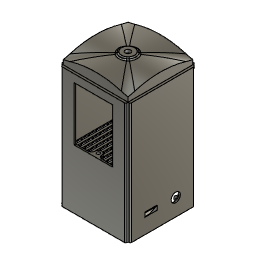
SolderingStation_Front (Autodesk Fusion 360 design; units mm, degrees)
Autodesk Fusion 360 part; units mm, degrees
sketch "Sketch1" plane through (0, 0, 0) normal (0, 0, 1) x (1, 0, 0)
  line L0 (45, 45) -> (-45, 45)
  line L1 (-45, 45) -> (-45, -45)
  line L2 (-45, -45) -> (45, -45)
  line L3 (45, -45) -> (45, 45)
  line L4 (45, 45) -> (-45, -45) construction
  line L5 (-45, 45) -> (45, -45) construction
  line L6 (0, 0) -> (0, -45) construction
  line L7 (0, 0) -> (-45, 0) construction
  line L8 (-45, -45) -> (-42, -45) construction
  line L9 (-42, -45) -> (-42, -42)
  line L10 (-45, -42) -> (-42, -42)
  line L11 (45, -42) -> (42, -42)
  line L12 (42, -45) -> (42, -42)
  line L13 (42, 45) -> (42, 42)
  line L14 (45, 42) -> (42, 42)
  line L15 (-45, 42) -> (-42, 42)
  line L16 (-42, 45) -> (-42, 42)
  dimension "d1" = 90
  dimension "d2" = 90
  dimension "d10" = 360
  constraint horizontal L0
  constraint perpendicular L0 L1
  constraint parallel L0 L2
  constraint parallel L1 L3
  constraint coincident L4 L6.start
  constraint coincident L5 L6.start
  constraint coincident L6.start L7.start
  constraint midpoint L2 L6.end
  constraint midpoint L1 L7.end
  constraint coincident L2 L8.end
  constraint coincident L4 L9.end
  constraint perpendicular L2 L9
  constraint perpendicular L9 L10
  measures "d1" distance of L1.end L2.end
  measures "d2" distance of L0.end L1.end
extrude "Extrude3" add sketch "Sketch1" along normal blind 2 contours L0 L1 L2 L3 L9 L10 L11 L12 L13 L14 L15 L16 makes body 1
sketch "Sketch3" plane through (0, 0, 0) normal (0, 0, -1) x (1, 0, 0)
  line L0 (-42, -45) -> (42, -45)
  line L1 (42, -45) -> (42, -42)
  line L2 (42, -42) -> (45, -42)
  line L3 (45, -42) -> (45, 42)
  line L4 (45, 42) -> (42, 42)
  line L5 (42, 42) -> (42, 45)
  line L6 (42, 45) -> (-42, 45)
  line L7 (-42, 45) -> (-42, 42)
  line L8 (-42, 42) -> (-45, 42)
  line L9 (-45, 42) -> (-45, -42)
  line L10 (-45, -42) -> (-42, -42)
  line L11 (-42, -42) -> (-42, -45)
  line L12 (43, -42) -> (43, 40)
  line L13 (43, 40) -> (40, 40)
  line L14 (40, 40) -> (40, 43)
  line L15 (40, 43) -> (-40, 43)
  line L16 (-40, 43) -> (-40, 40)
  line L17 (-40, 40) -> (-43, 40)
  line L18 (-43, 40) -> (-43, -42)
  line L19 (-45, -42) -> (-45, -40) construction
  line L20 (-45, -40) -> (-43, -40)
  line L21 (43, -40) -> (45, -40)
  dimension "d13" = -2
  constraint coincident L9.end L10.start
  constraint coincident L9 L19.end
  constraint perpendicular L10 L19
  constraint coincident L18 L20.end
  constraint perpendicular L18 L20
  constraint coincident L12 L21.start
  constraint coincident L3 L21.end
  constraint perpendicular L3 L21
extrude "Extrude4" add sketch "Sketch3" along normal blind 155 contours L3 L4 L5 L6 L7 L8 L9 L12 L13 L14 L15 L16 L17 L18 L20 L21 bodies 1
sketch "Sketch4" plane through (0, 40, 0) normal (0, 1, 0) x (-1, 0, 0)
  line L0 (45, 0) -> (43, 0)
  line L1 (43, 0) -> (43, -155)
  line L2 (43, -155) -> (45, -155)
  line L3 (45, -155) -> (45, 0)
  line L4 (43, -155) -> (43, -145) construction
  line L5 (43, -145) -> (37, -145) construction
  circle A0 centre (37, -145) radius 2.15
  circle A1 centre (37, -145) radius 4.5
  line L6 (37, -145) -> (37, -140.5) construction
  line L7 (37, -145) -> (37, -149.5) construction
  line L8 (37, -149.5) -> (43, -149.5)
  line L9 (37, -140.5) -> (43, -140.5)
  line L10 (0, -155) -> (0, 2) construction
  line L11 (-37, -140.5) -> (-43, -140.5)
  circle A2 centre (-37, -145) radius 4.5
  circle A3 centre (-37, -145) radius 2.15
  line L12 (-37, -149.5) -> (-43, -149.5)
  circle A4 centre (37, -5) radius 4.5
  circle A5 centre (37, -5) radius 2.15
  line L13 (37, -9.5) -> (43, -9.5)
  line L14 (37, -0.5) -> (43, -0.5)
  line L15 (-37, -0.5) -> (-43, -0.5)
  circle A6 centre (-37, -5) radius 4.5
  circle A7 centre (-37, -5) radius 2.15
  line L16 (-37, -9.5) -> (-43, -9.5)
  line L17 (-43, -140.5) -> (-43, -149.5)
  line L18 (-43, -0.5) -> (-43, -9.5)
  dimension "d16" = 4.3
  dimension "d17" = 9
  dimension "d18" = 4.3
  dimension "d19" = 9
  constraint coincident L1.end L2.start
  constraint coincident L1 L4.end
  constraint perpendicular L2 L4
  constraint perpendicular L4 L5
  constraint coincident L5.end A0.centre
  constraint concentric A0 A1
  constraint coincident A1 L6.end
  constraint perpendicular L5 L6
  constraint coincident A1 L7.end
  constraint perpendicular L5 L7
  constraint coincident L4 L8.end
  constraint coincident L1 L9.end
  constraint tangent A1 L9
  constraint perpendicular L9 L10
  constraint symmetric A0 L10 A3
  constraint symmetric A1 L10 A2
  constraint symmetric L6.end L10 L11.start
  constraint symmetric L7.end L10 L12.start
  constraint symmetric L8.end L10 L12.end
  constraint symmetric L9.end L10 L11.end
  constraint concentric A4 A5
  constraint coincident L14.start A4
  constraint coincident L13.start A4
  constraint tangent A4 L14
  constraint vertical L18
  measures "d16" diameter of A0
  measures "d17" diameter of A1
  measures "d18" diameter of A5
  measures "d19" diameter of A4
extrude "Extrude5" add sketch "Sketch4" against normal blind 13 contours L1 A4 L13 L14 | A4 | L1 A1 L8 L9 | A1 | L11 A2 L12 L17 | A2 | L15 A6 L16 L18 | A6 bodies 1
ref_plane "WorkPlane1" through (0, 35, 0) normal (0, 1, 0) x (0, 0, 1)
sketch "Sketch5" plane through (0, 35, 0) normal (0, 1, 0) x (1, 0, 0)
  circle A0 centre (37, 5) radius 2.15 construction
  line L0 (0, -2) -> (0, 155) construction
  line L1 (35.0226, 8.425) -> (33.0452, 5)
  line L2 (33.0452, 5) -> (35.0226, 1.575)
  line L3 (35.0226, 1.575) -> (38.9774, 1.575)
  line L4 (38.9774, 1.575) -> (40.9548, 5)
  line L5 (40.9548, 5) -> (38.9774, 8.425)
  line L6 (38.9774, 8.425) -> (35.0226, 8.425)
  line L7 (35.0226, 1.575) -> (31.6368, 1.575)
  line L8 (35.0226, 8.425) -> (31.5846, 8.425)
  line L9 (31.5846, 8.425) -> (31.6368, 1.575)
  line L10 (-35.0226, 1.575) -> (-38.9774, 1.575)
  line L11 (-38.9774, 1.575) -> (-40.9548, 5)
  line L12 (-40.9548, 5) -> (-38.9774, 8.425)
  line L13 (-38.9774, 8.425) -> (-35.0226, 8.425)
  line L14 (-35.0226, 8.425) -> (-31.5846, 8.425)
  line L15 (-31.5846, 8.425) -> (-31.6368, 1.575)
  line L16 (-35.0226, 1.575) -> (-31.6368, 1.575)
  line L17 (-33.0452, 5) -> (-35.0226, 1.575)
  line L18 (-35.0226, 8.425) -> (-33.0452, 5)
  line L19 (35.0226, 141.575) -> (38.9774, 141.575)
  line L20 (33.0452, 145) -> (35.0226, 141.575)
  line L21 (38.9774, 141.575) -> (40.9548, 145)
  line L22 (40.9548, 145) -> (38.9774, 148.425)
  line L23 (38.9774, 148.425) -> (35.0226, 148.425)
  line L24 (35.0226, 148.425) -> (31.5846, 148.425)
  line L25 (35.0226, 148.425) -> (33.0452, 145)
  line L26 (31.5846, 148.425) -> (31.6368, 141.575)
  line L27 (35.0226, 141.575) -> (31.6368, 141.575)
  line L28 (-38.9774, 141.575) -> (-40.9548, 145)
  line L29 (-35.0226, 141.575) -> (-38.9774, 141.575)
  line L30 (-35.0226, 141.575) -> (-31.6368, 141.575)
  line L31 (-31.5846, 148.425) -> (-31.6368, 141.575)
  line L32 (-35.0226, 148.425) -> (-31.5846, 148.425)
  line L33 (-35.0226, 148.425) -> (-33.0452, 145)
  line L34 (-33.0452, 145) -> (-35.0226, 141.575)
  line L35 (-38.9774, 148.425) -> (-35.0226, 148.425)
  line L36 (-40.9548, 145) -> (-38.9774, 148.425)
  point P0 (37, 5)
  dimension "d24" = 4.3
  dimension "d25" = 3.425
  constraint vertical L0
  constraint coincident P0 A0.centre
  constraint parallel L3 L7
  constraint parallel L6 L8
  constraint symmetric L0 L1.start L13.end
  constraint symmetric L0 L1.end L17.start
  constraint symmetric L0 L2.end L10.start
  constraint symmetric L0 L3.end L10.end
  constraint symmetric L0 L4.end L11.end
  constraint symmetric L0 L5.end L12.end
  constraint symmetric L0 L7.end L15.end
  constraint symmetric L0 L8.end L14.end
  constraint parallel L19 L27
  constraint parallel L23 L24
  measures "d24" diameter of A0
  measures "d25" distance of P0 L6
extrude "Extrude6" cut sketch "Sketch5" against normal blind 3 bodies 1
sketch "Sketch6" plane through (0, -45, 0) normal (0, -1, 0) x (1, 0, 0)
  line L0 (42, -155) -> (42, 2)
  line L1 (42, 2) -> (-42, 2)
  line L2 (-42, 2) -> (-42, -155)
  line L3 (-42, -155) -> (42, -155)
  line L4 (0, 2) -> (0, -155) construction
  line L5 (25, -8) -> (-25, -8)
  line L6 (-25, -8) -> (-25, -78)
  line L7 (-25, -78) -> (25, -78)
  line L8 (25, -78) -> (25, -8)
  line L9 (25, -8) -> (-25, -78) construction
  line L10 (-25, -8) -> (25, -78) construction
  point P0 (0, -43)
  dimension "d28" = 70
  dimension "d29" = 50
  dimension "d30" = 45
  constraint midpoint L1 L4.start
  constraint midpoint L3 L4.end
  constraint horizontal L5
  constraint perpendicular L5 L6
  constraint parallel L5 L7
  constraint parallel L6 L8
  constraint coincident L9 P0
  constraint coincident L10 P0
  constraint coincident L4 P0
  measures "d28" distance of L5.start L7.end
  measures "d29" distance of L5.start L5.end
  measures "d30" distance of L1 P0
extrude "Extrude7" cut sketch "Sketch6" against normal blind 2 contours L5 L6 L7 L8 bodies 1
sketch "Sketch7" plane through (0, -45, 0) normal (0, -1, 0) x (1, 0, 0)
  line L0 (-25, -8) -> (25, -8)
  line L1 (25, -8) -> (25, -78)
  line L2 (25, -78) -> (-25, -78)
  line L3 (-25, -78) -> (-25, -8)
  line L4 (42, -155) -> (42, 2)
  line L5 (42, 2) -> (-42, 2)
  line L6 (-42, 2) -> (-42, -155)
  line L7 (-42, -155) -> (42, -155)
  line L8 (0, 2) -> (0, -155) construction
  line L9 (4.5, -8) -> (-4.5, -8)
  line L10 (-4.5, -8) -> (-4.5, -5)
  line L11 (-4.5, -5) -> (4.5, -5)
  line L12 (4.5, -5) -> (4.5, -8)
  line L13 (25, -43) -> (-25, -43) construction
  line L14 (-4.5, -81) -> (4.5, -81)
  line L15 (4.5, -78) -> (-4.5, -78)
  line L16 (-4.5, -78) -> (-4.5, -81)
  line L17 (4.5, -81) -> (4.5, -78)
  dimension "d35" = 9
  dimension "d36" = 3
  dimension "d37" = 4.5
  constraint midpoint L5 L8.start
  constraint midpoint L7 L8.end
  constraint horizontal L9
  constraint vertical L10
  constraint horizontal L11
  constraint vertical L12
  constraint midpoint L1 L13.start
  constraint midpoint L3 L13.end
  constraint symmetric L9.start L13 L15.start
  constraint symmetric L9.end L13 L15.end
  constraint symmetric L10.end L13 L14.start
  constraint symmetric L11.end L13 L14.end
  measures "d35" distance of L9.start L9.end
  measures "d36" distance of L9.start L11.end
  measures "d37" distance of L8 L12
extrude "Extrude8" add sketch "Sketch7" against normal blind 11 contours L0 L9 L10 L11 L12 | L2 L14 L15 L16 L17 bodies 1
sketch "Sketch9" plane through (0, 0, -81) normal (0, 0, -1) x (1, 0, 0)
  line L0 (4.5, 43) -> (-4.5, 43)
  line L1 (-4.5, 43) -> (-4.5, 34)
  line L2 (-4.5, 34) -> (4.5, 34)
  line L3 (4.5, 34) -> (4.5, 43)
  line L4 (-4.5, 43) -> (4.5, 34) construction
  line L5 (-4.5, 34) -> (4.5, 43) construction
  circle A0 centre (0, 38.5) radius 2.15
  dimension "d40" = 4.3
  constraint coincident L0.end L1.start
  constraint coincident L2.end L3.start
  constraint coincident L1.end L2.start
  constraint coincident L0.start L3.end
  constraint midpoint L5 A0.centre
  measures "d40" diameter of A0
extrude "Extrude9" cut sketch "Sketch9" against normal blind 80 contours A0 bodies 1
fillet "Fillet1" radius 4.5 8 edges at (4.5, -34, -79.5) (-4.5, -34, -79.5) (4.5, -43, -79.5) (-4.5, -43, -79.5) (4.5, -34, -6.5) (-4.5, -34, -6.5) (4.5, -43, -6.5) (-4.5, -43, -6.5) on bodies 1
sketch "Sketch10" plane through (0, 0, -155) normal (0, 0, -1) x (1, 0, 0)
  line L0 (43, 40) -> (43, -40)
  line L1 (43, -40) -> (45, -40)
  line L2 (45, -40) -> (45, 42)
  line L3 (45, 42) -> (42, 42)
  line L4 (42, 42) -> (42, 45)
  line L5 (42, 45) -> (-42, 45)
  line L6 (-42, 45) -> (-42, 42)
  line L7 (-42, 42) -> (-45, 42)
  line L8 (-45, 42) -> (-45, -40)
  line L9 (-45, -40) -> (-43, -40)
  line L10 (-43, -40) -> (-43, 40)
  line L11 (-43, 40) -> (-40, 40)
  line L12 (-40, 40) -> (-40, 43)
  line L13 (-40, 43) -> (40, 43)
  line L14 (40, 43) -> (40, 40)
  line L15 (40, 40) -> (43, 40)
  line L16 (0, 0) -> (0, 45) construction
  circle A0 centre (-36.452, 36.452) radius 2.15
  circle A1 centre (-36.452, 36.452) radius 4.5
  line L17 (-36.452, 36.452) -> (-31.952, 36.452) construction
  line L18 (-36.452, 36.452) -> (-36.452, 31.952) construction
  line L19 (-31.952, 36.452) -> (-31.952, 45)
  line L20 (-36.452, 31.952) -> (-45, 31.952)
  line L21 (31.952, 36.452) -> (31.952, 45)
  circle A2 centre (36.452, 36.452) radius 4.5
  circle A3 centre (36.452, 36.452) radius 2.15
  line L22 (36.452, 31.952) -> (45, 31.952)
  dimension "d45" = 4.3
  dimension "d46" = 8.548
  dimension "d47" = 8.548
  dimension "d48" = 9
  constraint coincident L16.start origin
  constraint midpoint L5 L16.end
  constraint concentric A0 A1
  constraint coincident A0.centre A1.centre
  constraint coincident A1 L17.end
  constraint parallel L13 L17
  constraint coincident A1 L18.end
  constraint perpendicular L17 L18
  constraint coincident L5 L19.end
  constraint tangent A1 L19
  constraint tangent A1 L20
  constraint symmetric L16 A0 A3
  constraint symmetric L16 A1 A2
  constraint symmetric L16 L17.end L21.start
  constraint symmetric L16 L18.end L22.start
  constraint symmetric L16 L19.end L21.end
  constraint symmetric L16 L20.end L22.end
  measures "d45" diameter of A0
  measures "d46" distance of L5 A0.centre
  measures "d47" distance of L8 A0.centre
  measures "d48" diameter of A1
extrude "Extrude10" add sketch "Sketch10" against normal blind 13 contours L0 L13 L14 L15 L21 A2 L22 | A2 | L10 L11 L12 L13 A1 L19 L20 | A1 bodies 1
ref_plane "WorkPlane2" through (0, 0, -150) normal (0, 0, 1) x (1, 0, 0)
sketch "Sketch11" plane through (0, 0, -150) normal (0, 0, 1) x (1, 0, 0)
  circle A0 centre (-36.454, -36.454) radius 2.15 construction
  line L0 (42, -45) -> (-42, -45) construction
  line L1 (-45, -42) -> (-45, 40) construction
  line L2 (0, -45) -> (0, 0) construction
  line L3 (-39.879, -38.4314) -> (-36.454, -40.4088)
  line L4 (-36.454, -40.4088) -> (-33.029, -38.4314)
  line L5 (-33.029, -38.4314) -> (-33.029, -34.4766)
  line L6 (-33.029, -34.4766) -> (-36.454, -32.4992)
  line L7 (-36.454, -32.4992) -> (-39.879, -34.4766)
  line L8 (-39.879, -34.4766) -> (-39.879, -38.4314)
  line L9 (-39.879, -34.4766) -> (-39.879, -31.1512)
  line L10 (-33.029, -34.4766) -> (-33.029, -31)
  line L11 (-33.029, -31) -> (-39.879, -31.1512)
  line L12 (33.029, -38.4314) -> (33.029, -34.4766)
  line L13 (36.454, -40.4088) -> (33.029, -38.4314)
  line L14 (39.879, -38.4314) -> (36.454, -40.4088)
  line L15 (39.879, -34.4766) -> (39.879, -38.4314)
  line L16 (36.454, -32.4992) -> (39.879, -34.4766)
  line L17 (33.029, -34.4766) -> (36.454, -32.4992)
  line L18 (33.029, -31) -> (39.879, -31.1512)
  line L19 (33.029, -34.4766) -> (33.029, -31)
  line L20 (39.879, -34.4766) -> (39.879, -31.1512)
  point P0 (-36.454, -36.454)
  dimension "d52" = 4.3
  dimension "d53" = 8.546
  dimension "d54" = 8.546
  dimension "d55" = 3.425
  constraint midpoint L0 L2.start
  constraint coincident L2.end origin
  constraint coincident P0 A0.centre
  constraint parallel L8 L9
  constraint parallel L5 L10
  constraint symmetric L2 L3.start L14.start
  constraint symmetric L2 L3.end L13.start
  constraint symmetric L2 L4.end L12.start
  constraint symmetric L2 L5.end L12.end
  constraint symmetric L2 L6.end L16.start
  constraint symmetric L2 L7.end L15.start
  constraint symmetric L2 L9.end L18.end
  constraint symmetric L2 L10.end L18.start
  measures "d52" diameter of A0
  measures "d53" distance of P0 L0
  measures "d54" distance of P0 L1
  measures "d55" distance of P0 L8
extrude "Extrude11" cut sketch "Sketch11" against normal blind 3 bodies 1
ref_plane "WorkPlane3" through (0, -25, 0) normal (0, 1, 0) x (0, 0, 1)
sketch "Sketch13" plane through (0, -25, 0) normal (0, 1, 0) x (1, 0, 0)
  line L0 (43, 138.3124) -> (37.453, 146.6329)
  line L1 (43, 138.3124) -> (53, 138.3124) construction
  line L2 (37.453, 146.6329) -> (34.7904, 144.8578)
  line L3 (43, 138.3124) -> (43, 124) construction
  line L4 (34.7904, 144.8578) -> (43, 132.5435)
  line L5 (44.6641, 139.4218) -> (38.0077, 149.4064)
  line L6 (38.0077, 149.4064) -> (32.0169, 145.4125)
  line L7 (32.0169, 145.4125) -> (41.3359, 131.4341)
  line L8 (41.3359, 131.4341) -> (43, 128.9379)
  line L9 (43, 138.3124) -> (43, 151) construction
  line L10 (38.0077, 149.4064) -> (43, 149.4064)
  line L11 (43, 128.9379) -> (43, 141.9179)
  line L12 (38.0077, 149.4064) -> (43, 141.9179)
  line L13 (43, 141.9179) -> (43, 149.4064)
  line L14 (37.453, 146.6329) -> (36.3436, 148.297)
  line L15 (34.7904, 144.8578) -> (33.681, 146.5219)
  dimension "d59" = 123.69
  dimension "d60" = 10
  dimension "d61" = 3.2
  dimension "d62" = 2
  constraint horizontal L1
  constraint perpendicular L0 L2
  constraint perpendicular L1 L3
  constraint coincident L3 L4.end
  constraint perpendicular L2 L4
  constraint coincident L3 L8.end
  constraint parallel L7 L8
  constraint perpendicular L1 L9
  constraint coincident L9 L10.end
  constraint perpendicular L9 L10
  constraint coincident L9 L11.end
  constraint coincident L5 L11.end
  constraint coincident L6 L14.end
  constraint perpendicular L6 L14
  constraint coincident L6 L15.end
  constraint perpendicular L6 L15
  measures "d59" angle of L0 L1
  measures "d60" distance of L0.start L0.end
  measures "d61" distance of L0.end L2.end
extrude "Extrude12" add sketch "Sketch13" along normal blind 18 contours L0 L5 L6 L11 L12 L14 | L4 L6 L7 L8 L11 L15 | L5 L10 L12 L13 bodies 1
sketch "Sketch14" plane through (0, -25, 0) normal (0, -1, 0) x (1, 0, 0)
  line L0 (43, -149.4064) -> (43, -138.3124)
  line L1 (43, -138.3124) -> (36.3436, -148.297)
  line L2 (33.681, -146.5219) -> (43, -132.5435)
  line L3 (43, -132.5435) -> (43, -128.9379)
  line L4 (43, -128.9379) -> (32.0169, -145.4125)
  line L5 (32.0169, -145.4125) -> (33.681, -146.5219)
  line L6 (38.0077, -149.4064) -> (43, -149.4064)
  line L7 (43, -128.9379) -> (43, -149.4064)
  line L8 (38.0077, -149.4064) -> (43, -149.4064)
  line L9 (38.0077, -149.4064) -> (32.0169, -145.4125)
  line L10 (32.0169, -145.4125) -> (43, -128.9379)
  line L11 (37.453, -146.6329) -> (36.3436, -148.297)
  line L12 (34.7904, -144.8578) -> (33.681, -146.5219)
  line L13 (36.3436, -148.297) -> (38.0077, -149.4064)
  constraint coincident L3.end L4.start
  constraint coincident L0.start L6.end
  constraint coincident L2.start L6.start
  constraint coincident L4.end L5.start
  constraint coincident L1.end L11.start
  constraint coincident L9 L1.end
  constraint perpendicular L9 L11
  constraint coincident L2.start L12.start
  constraint coincident L9 L2.start
  constraint perpendicular L9 L12
extrude "Extrude13" add sketch "Sketch14" against normal blind 2 separate body contours L1 L2 L7 L9 L11 L12 | L2 L3 L4 L5 L7 L9 L10 L12 makes body 2
combine "Combine1" operation add target body 2 tool bodies 1
sketch "Sketch15" plane through (0, -7, 0) normal (0, 1, 0) x (-1, 0, 0)
  line L0 (-43, -138.3124) -> (-43, -149.4064)
  line L1 (-43, -149.4064) -> (-38.0077, -149.4064)
  line L2 (-33.681, -146.5219) -> (-32.0169, -145.4125)
  line L3 (-32.0169, -145.4125) -> (-43, -128.9379)
  line L4 (-43, -128.9379) -> (-43, -132.5435)
  line L5 (-43, -132.5435) -> (-33.681, -146.5219)
  line L6 (-36.3436, -148.297) -> (-43, -138.3124)
  line L7 (-43, -128.9379) -> (-43, -149.4064)
  line L8 (-33.681, -146.5219) -> (-32.0169, -145.4125)
  line L9 (-32.0169, -145.4125) -> (-43, -128.9379)
  line L10 (-38.0077, -149.4064) -> (-36.3436, -148.297)
  line L11 (-38.0077, -149.4064) -> (-33.681, -146.5219)
  constraint coincident L3.end L4.start
  constraint coincident L0.end L1.start
  constraint coincident L2.start L5.end
  constraint coincident L2.end L3.start
  constraint coincident L1.end L10.start
extrude "Extrude14" add sketch "Sketch15" along normal blind 2 bodies 2
fillet "Fillet2" radius 4 1 edges at (32.0169, -15, -145.4125) on bodies 2
ref_plane "WorkPlane4" through (0, -23, 0) normal (0, 1, 0) x (0, 0, 1)
sketch "Sketch17" plane through (0, -23, 0) normal (0, 1, 0) x (1, 0, 0)
  line L0 (42.5, 133.3) -> (45.2735, 129.1397)
  line L1 (42.5, 133.3) -> (47.5, 133.3) construction
  line L2 (34.7904, 144.8578) -> (43, 132.5435)
  line L3 (42.7331, 138.7127) -> (46.6535, 132.8321)
  line L4 (43, 138.3124) -> (37.453, 146.6329)
  line L5 (46.6535, 132.8321) -> (45.2735, 129.1397)
  line L6 (42.5, 133.3) -> (42.7331, 138.7127)
  dimension "d73" = 5
  constraint horizontal L1
  constraint parallel L0 L2
  constraint parallel L3 L4
  constraint coincident L3.start L4
  measures "d73" distance of L0.start L0.end
extrude "Extrude15" cut sketch "Sketch17" along normal blind 16 bodies 2
sketch "Sketch18" plane through (0, -5, 0) normal (0, 1, 0) x (-1, 0, 0)
  arc A0 (-35.3451, -147.6313) -> (-34.2357, -142.0843) centre (-37.5639, -144.3031) ccw
  line L0 (-34.2357, -142.0843) -> (-43, -128.9379)
  line L1 (-43, -128.9379) -> (-43, -149.4064)
  line L2 (-34.2357, -142.0843) -> (-35.3451, -147.6313)
  line L3 (-38.0077, -149.4064) -> (-35.3451, -147.6313)
  line L4 (-43, -149.4064) -> (-38.0077, -149.4064)
  constraint coincident A0.end L0.start
  constraint coincident A0.start L2.end
extrude "Extrude16" cut sketch "Sketch18" against normal blind 21 contours A0 L2 bodies 2
sketch "Sketch20" plane through (45, 0, 0) normal (1, 0, 0) x (0, 1, 0)
  line L0 (-7, -135.3124) -> (-23, -135.3124)
  line L1 (-23, -135.3124) -> (-23, -129.55)
  line L2 (-23, -129.55) -> (-7, -129.55)
  line L3 (-7, -129.55) -> (-7, -135.3124)
  line L4 (40, 0) -> (42, 0)
  line L5 (42, 0) -> (42, 2)
  line L6 (42, 2) -> (-42, 2)
  line L7 (-42, 2) -> (-42, -155)
  line L8 (-42, -155) -> (40, -155)
  line L9 (40, -155) -> (40, 0)
  circle A0 centre (17, -133) radius 6
  dimension "d78" = 12
  measures "d78" diameter of A0
extrude "Extrude17" cut sketch "Sketch20" against normal blind 2 contours A0 bodies 2
ref_plane "WorkPlane5" through (0, -25, 0) normal (0, 1, 0) x (0, 0, 1)
sketch "Sketch23" plane through (0, -25, 0) normal (0, 1, 0) x (1, 0, 0)
  line L0 (-43, 114) -> (-45, 114)
  line L1 (-43, 114) -> (-43, 132.4964) construction
  line L2 (-45, 114) -> (-43, 110.5359)
  line L3 (-45, 114) -> (-41, 114) construction
  line L4 (-45, 135) -> (-43, 131.5359)
  line L5 (-45, 129) -> (-43, 125.5359)
  line L6 (-45, 132) -> (-43, 128.5359)
  line L7 (-45, 126) -> (-43, 122.5359)
  line L8 (-45, 123) -> (-43, 119.5359)
  line L9 (-45, 120) -> (-43, 116.5359)
  line L10 (-45, 117) -> (-43, 113.5359)
  line L11 (-45, 114) -> (-43, 110.5359)
  line L12 (-45, 111) -> (-43, 107.5359)
  line L13 (-45, 108) -> (-43, 104.5359)
  line L14 (-45, 105) -> (-43, 101.5359)
  line L15 (-45, 102) -> (-43, 98.5359)
  line L16 (-45, 99) -> (-43, 95.5359)
  line L17 (-45, 96) -> (-43, 92.5359)
  line L18 (-45, 93) -> (-43, 89.5359)
  line L19 (-43, 135) -> (-43, 89.5359)
  line L20 (-43, 89.5359) -> (-45, 89.5359)
  line L21 (-45, 89.5359) -> (-45, 135)
  line L22 (-45, 147) -> (-43, 143.5359)
  line L23 (-45, 144) -> (-43, 140.5359)
  line L24 (-45, 141) -> (-43, 137.5359)
  line L25 (-45, 138) -> (-43, 134.5359)
  line L26 (-45, 147) -> (-43, 147)
  line L27 (-43, 147) -> (-43, 135)
  line L28 (-45, 147) -> (-45, 138)
  line L29 (-45, 138) -> (-45, 135)
  dimension "d89" = 60
  constraint horizontal L0
  constraint perpendicular L0 L1
  constraint horizontal L3
  constraint coincident L1 L2.end
  constraint perpendicular L19 L20
  constraint horizontal L26
  constraint perpendicular L26 L27
  constraint perpendicular L26 L28
  constraint parallel L21 L29
  measures "d89" angle of L2 L3
extrude "Extrude21" cut sketch "Sketch23" along normal blind 50 contours L0 L2 L10 L11 L19 | L0 L10 L21 | L8 L9 L19 L21 | L12 L13 L19 L21 | L5 L7 L19 L21 | L14 L15 L19 L21 | L4 L6 L19 L21 | L16 L17 L19 L21 | L19 L24 L25 L27 L28 | L22 L23 L27 L28 bodies 2
sketch "Sketch24" plane through (0, 0, 2) normal (0, 0, 1) x (-1, 0, 0)
  line L0 (-42, -45) -> (42, -45)
  line L1 (42, -45) -> (42, -42)
  line L2 (42, -42) -> (45, -42)
  line L3 (45, -42) -> (45, 42)
  line L4 (45, 42) -> (42, 42)
  line L5 (42, 42) -> (42, 45)
  line L6 (42, 45) -> (-42, 45)
  line L7 (-42, 45) -> (-42, 42)
  line L8 (-42, 42) -> (-45, 42)
  line L9 (-45, 42) -> (-45, -42)
  line L10 (-45, -42) -> (-42, -42)
  line L11 (-42, -42) -> (-42, -45)
  line L12 (42, -42) -> (-42, -42)
  line L13 (-42, -42) -> (-42, 42)
  line L14 (-42, 42) -> (42, 42)
  line L15 (42, 42) -> (42, -42)
  constraint horizontal L12
  constraint vertical L13
  constraint horizontal L14
  constraint vertical L15
  constraint coincident L7.end L8.start
  constraint coincident L1.end L2.start
extrude "Extrude22" add sketch "Sketch24" along normal blind 5 contours L12 L13 L14 L15 bodies 2
sketch "Sketch25" plane through (0, 0, 7) normal (0, 0, 1) x (-1, 0, 0)
  line L0 (42, 42) -> (-42, 42)
  line L1 (-42, 42) -> (-42, -42)
  line L2 (-42, -42) -> (42, -42)
  line L3 (42, -42) -> (42, 42)
  line L4 (-40, 40) -> (-40, -40)
  line L5 (-40, -40) -> (40, -40)
  line L6 (40, -40) -> (40, 40)
  line L7 (40, 40) -> (-40, 40)
  dimension "d98" = -2
extrude "Extrude23" cut sketch "Sketch25" against normal blind 7 contours L4 L5 L6 L7 bodies 2
fillet "Fillet3" radius 1.5 12 edges at (-45, -42, -76.5) (-42, -42, -76.5) (-42, -45, -76.5) (42, -42, -76.5) (42, -45, -76.5) (45, -42, -76.5) (45, 42, 1) (42, 42, 1) (42, 45, 1) (-42, 45, 1) (-42, 42, 1) (-45, 42, 1) on bodies 2
sketch "Sketch27" plane through (0, 0, 7) normal (0, 0, 1) x (-1, 0, 0)
  line L0 (-40, -40) -> (-40, 40)
  line L1 (-40, 40) -> (40, 40)
  line L2 (40, 40) -> (40, -40)
  line L3 (40, -40) -> (-40, -40)
  line L4 (42, 42) -> (-42, 42)
  line L5 (-42, 42) -> (-42, -42)
  line L6 (-42, -42) -> (42, -42)
  line L7 (42, -42) -> (42, 42)
  line L8 (42, -42) -> (-42, -42)
  line L9 (-42, -42) -> (-42, 42)
  line L10 (-42, 42) -> (42, 42)
  line L11 (42, 42) -> (42, -42)
  constraint horizontal L8
  constraint vertical L9
  constraint horizontal L10
  constraint vertical L11
  constraint coincident L4.end L5.start
  constraint coincident L6.end L7.start
ref_plane "WorkPlane6" through (0, 0, 10) normal (0, 0, 1) x (1, 0, 0)
sketch "Sketch29" plane through (0, -42, 0) normal (0, -1, 0) x (1, 0, 0)
  line L0 (-42, 2) -> (42, 2)
  line L1 (42, 2) -> (42, 7)
  line L2 (42, 7) -> (-42, 7)
  line L3 (-42, 7) -> (-42, 2)
  arc A0 (42, 7) -> (-42, 7) centre (0, -100.0561) ccw
  dimension "d127" = 115
  constraint coincident L1.end L2.start
  constraint coincident L2.end L3.start
  measures "d127" radius of A0
sketch "Sketch30" plane through (42, 0, 0) normal (1, 0, 0) x (0, 1, 0)
  line L0 (-42, 2) -> (42, 2)
  line L1 (42, 2) -> (42, 7)
  line L2 (42, 7) -> (-42, 7)
  line L3 (-42, 7) -> (-42, 2)
  arc A0 (42, 7) -> (-42, 7) centre (0, -100.0561) ccw
  dimension "d128" = 115
  constraint coincident L1.end L2.start
  constraint coincident L2.end L3.start
  measures "d128" radius of A0
sketch "Sketch31" plane through (0, 42, 0) normal (0, 1, 0) x (-1, 0, 0)
  line L0 (-42, 2) -> (42, 2)
  line L1 (42, 2) -> (42, 7)
  line L2 (42, 7) -> (-42, 7)
  line L3 (-42, 7) -> (-42, 2)
  arc A0 (42, 7) -> (-42, 7) centre (0, -100.0561) ccw
  dimension "d129" = 115
  constraint coincident L1.end L2.start
  constraint coincident L2.end L3.start
  measures "d129" radius of A0
sketch "Sketch32" plane through (-42, 0, 0) normal (-1, 0, 0) x (0, -1, 0)
  line L0 (-42, 2) -> (42, 2)
  line L1 (42, 2) -> (42, 7)
  line L2 (42, 7) -> (-42, 7)
  line L3 (-42, 7) -> (-42, 2)
  arc A0 (42, 7) -> (-42, 7) centre (0, -100.0561) ccw
  dimension "d130" = 115
  constraint coincident L1.end L2.start
  constraint coincident L2.end L3.start
  measures "d130" radius of A0
extrude "Extrude24" add sketch "Sketch32" against normal blind 84 contours L2 A0 bodies 2
extrude "Extrude25" add sketch "Sketch31" against normal blind 84 contours L2 A0 bodies 2
sketch "Sketch33" plane through (0, 0, 7) normal (0, 0, 1) x (1, 0, 0)
  circle A0 centre (0, 0) radius 10
  dimension "d106" = 20
  constraint coincident A0.centre origin
  measures "d106" diameter of A0
extrude "Extrude26" add sketch "Sketch33" along normal blind 10 bodies 2
fillet "Fillet4" radius 30 4 edges at (-21.3723, -21.3723, 12.9405) (21.3723, -21.3723, 12.9405) (21.3723, 21.3723, 12.9405) (-21.3723, 21.3723, 12.9405) on bodies 2
fillet "Fillet5" radius 2 15 edges at (-7.0711, -7.0711, 14.7515) (7.0711, 7.0711, 14.7515) (10, 0, 14.9439) (7.0711, -7.0711, 14.7515) (0, -10, 14.9439) (0, 10, 14.9439) (-7.0711, -7.0711, 14.7515) (7.0711, 7.0711, 14.7515) (-10, 0, 14.9439) (10, 0, 14.9439) (7.0711, -7.0711, 14.7515) (-7.0711, 7.0711, 14.7515) (0, -10, 14.9439) (0, 10, 14.9439) (-9.3233, -3.6162, 17) on bodies 2
sketch "Sketch35" plane through (0, 0, 7) normal (0, 0, 1) x (1, 0, 0)
  line L0 (-10, 10) -> (10, 10)
  line L1 (10, 10) -> (10, -10)
  line L2 (10, -10) -> (-10, -10)
  line L3 (-10, -10) -> (-10, 10)
  line L4 (-10, 10) -> (10, -10) construction
  line L5 (10, 10) -> (-10, -10) construction
  dimension "d114" = 20
  dimension "d115" = 20
  constraint horizontal L0
  constraint perpendicular L0 L1
  constraint parallel L0 L2
  constraint parallel L1 L3
  constraint coincident L4 origin
  constraint coincident L5 origin
  measures "d114" distance of L1.end L2.end
  measures "d115" distance of L0.end L1.end
extrude "Extrude27" cut sketch "Sketch35" along normal blind 6 bodies 2
sketch "Sketch36" plane through (0, 0, 17) normal (0, 0, 1) x (-1, 0, 0)
  circle A0 centre (0, 0) radius 3.5
  spline S0 degree 3 poles (-6.5759, -5.1963) (-6.9367, -4.7701) (-7.2575, -4.3039) (-7.9165, -3.0947) (-8.1977, -2.3236) (-8.4546, -1.0183) (-8.5041, -0.5069) (-8.5041, 0) (-8.5041, 0.5069) (-8.4546, 1.0184) (-8.1977, 2.3237) (-7.9165, 3.0948) (-7.2574, 4.304) (-6.9367, 4.7702) (-6.5759, 5.1963) knots 0 0 0 0 0.167511 0.167511 0.410806 0.410806 0.562865 0.562865 0.562865 0.714929 0.714929 0.958231 0.958231 1.12573 1.12573 1.12573 1.12573
  spline S1 degree 3 poles (-5.1963, -6.5759) (-5.4447, -6.3656) (-5.6846, -6.1449) (-6.1449, -5.6846) (-6.3656, -5.4447) (-6.5759, -5.1963) knots 0 0 0 0 0.097638 0.097638 0.195275 0.195275 0.195275 0.195275
  spline S2 degree 3 poles (5.1963, -6.5759) (4.5268, -7.1427) (3.7669, -7.6046) (2.1233, -8.2633) (1.2434, -8.4554) (-0.7983, -8.549) (-1.9726, -8.3396) (-3.8244, -7.5687) (-4.5571, -7.117) (-5.1963, -6.5759) knots 0 0 0 0 0.26314 0.26314 0.527498 0.527498 0.873988 0.873988 1.125236 1.125236 1.125236 1.125236
  spline S3 degree 3 poles (6.5759, -5.1963) (6.3656, -5.4447) (6.1449, -5.6846) (5.6846, -6.1449) (5.4447, -6.3656) (5.1963, -6.5759) knots 0 0 0 0 0.097638 0.097638 0.195275 0.195275 0.195275 0.195275
  spline S4 degree 3 poles (6.5759, 5.1963) (7.117, 4.5571) (7.5687, 3.8244) (8.3396, 1.9726) (8.549, 0.7983) (8.4554, -1.2434) (8.2633, -2.1233) (7.6046, -3.7669) (7.1427, -4.5268) (6.5759, -5.1963) knots 0 0 0 0 0.251248 0.251248 0.597738 0.597738 0.862096 0.862096 1.125236 1.125236 1.125236 1.125236
  spline S5 degree 3 poles (5.1963, 6.5759) (5.4447, 6.3656) (5.6846, 6.1449) (6.1449, 5.6846) (6.3656, 5.4447) (6.5759, 5.1963) knots 0 0 0 0 0.097638 0.097638 0.195275 0.195275 0.195275 0.195275
  spline S6 degree 3 poles (-5.1963, 6.5759) (-4.5571, 7.117) (-3.8244, 7.5687) (-1.9726, 8.3396) (-0.7983, 8.549) (1.2434, 8.4554) (2.1234, 8.2633) (3.7669, 7.6046) (4.5269, 7.1426) (5.1963, 6.5759) knots 0 0 0 0 0.251248 0.251248 0.597739 0.597739 0.862101 0.862101 1.125237 1.125237 1.125237 1.125237
  spline S7 degree 3 poles (-6.5759, 5.1963) (-6.3656, 5.4447) (-6.1449, 5.6846) (-5.6846, 6.1449) (-5.4447, 6.3656) (-5.1963, 6.5759) knots 0 0 0 0 0.097638 0.097638 0.195275 0.195275 0.195275 0.195275
  dimension "d118" = 7
  constraint coincident A0.centre origin
  measures "d118" diameter of A0
extrude "Extrude28" cut sketch "Sketch36" against normal blind 5 contours A0 bodies 2
ref_plane "WorkPlane7" through (0, 0, 0) normal (0, 0, 1) x (1, 0, 0)
sketch "Sketch38" plane through (0, 0, 0) normal (0, 0, 1) x (1, 0, 0)
  line L0 (-9, -43) -> (9, -43)
  line L1 (9, -43) -> (9, -31)
  line L2 (9, -31) -> (-9, -31)
  line L3 (-9, -31) -> (-9, -43)
  dimension "d124" = 12
  constraint horizontal L0
  constraint vertical L1
  constraint horizontal L2
  constraint vertical L3
  measures "d124" distance of L0.end L1.end
extrude "Extrude29" add sketch "Sketch38" along normal blind 9 bodies 2
extrude "Extrude30" cut 1 faces at (-9, -42.6667, 6) along direction (1, 0, 0) blind 18 on bodies 2 bodies 2
equation "d20 = -5 mm - 3 mm - 5 mm"
equation "d23 = 45 mm - 5 mm - 5 mm"
equation "d49 = -5 mm - 3 mm - 5 mm"
equation "d51 = -155.00 mm + 5 mm"
equation "d59 = 33.69 deg + 90 deg"
